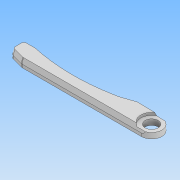
# Autodesk Inventor part: DoubleCrossBar
Saved by Autodesk Inventor 2021 (Build 250183000, 183)
## iProperties
Created: 2021-02-18
Part Number: DoubleCrossBar
Material: 一般
Document SubType Name: Modeling
Designer: kumagai
Density: 1 g/cm^3
Appearance: 既定
Author: kumagai
Autodesk Inventor part; units mm, degrees
ref_plane "YZ Plane" through (0, 0, 0) normal (1, 0, 0) x (0, 1, 0)
ref_plane "XZ Plane" through (0, 0, 0) normal (0, 1, 0) x (-1, 0, 0)
ref_plane "XY Plane" through (0, 0, 0) normal (0, 0, 1) x (1, 0, 0)
sketch "スケッチ1" plane through (0, 0, 0) normal (0, 1, 0) x (-1, 0, 0)
  line L0 (0, -94.2305) -> (0, 20.4332) projected
  line L1 (-15.3636, 0) -> (63.8106, 0) projected
  arc A0 (0, 4) -> (-0.1067, -3.9986) centre (0, 0) ccw
  line L2 (0, 4) -> (46.9019, 4)
  arc A1 (47.548, -2.5) -> (16.9578, -1.985) centre (30.98, -77.85) ccw
  line L3 (52.5, 2.5) -> (52.5, -2.5)
  line L4 (-0.1067, -3.9986) -> (9.3002, -4.2495)
  circle A2 centre (0, 0) radius 2.55
  line L5 (52.5, 2.5) -> (46.9019, 4)
  line L6 (52.5, -2.5) -> (47.548, -2.5)
  line L7 (9.3002, -4.2495) -> (14.9911, -2.3485)
  line L8 (14.9911, -2.3485) -> (16.9578, -1.985)
  dimension "d1" = 8
  dimension "d2" = 81.85
  dimension "d5" = 5.1
  dimension "d12" = 2.5
  dimension "d13" = 2.5
  dimension "d14" = 15
  dimension "d16" = 52.5
  dimension "d17" = 21.52
  dimension "d23" = 20
  dimension "d24" = 2
  dimension "d25" = 8
  dimension "d26" = 6
  dimension "d27" = 77.15
  constraints: 14 end point, 4 point on circle, 3 centre point, 3 tangent, 2 coincident, 2 horizontal, 1 point on line, 1 vertical
  measures "d1" diameter of A0
  measures "d2" distance from line of A1.centre L2
  measures "d5" diameter of A2
  measures "d12" distance between parallel lines of L6 L1
  measures "d13" distance from line of L1 L3.start
  measures "d14" angle of L2 L5
  measures "d16" distance between parallel lines of L3 L0
  measures "d17" distance from line of A1.centre L3
  measures "d23" angle of L4 L7
  measures "d24" distance of L7.end L8.end
  measures "d25" angle of L7 L8
  measures "d26" distance of L4.end L7.end
  measures "d27" radius of A1
extrude "押し出し1" add sketch "スケッチ1" along normal blind 3.2 contours L4 A0 L1 A2 L0 | L0 A2 L1 L3 L6 A1 L8 L7 L4 | L1 A0 L0 A2 | A2 L0 L2 L5 L3 L1
fillet "フィレット1" radius 1.5 6 edges at (-52.5, 1.6, 2.5) (-46.9019, 1.6, 4) (-52.5, 1.6, -2.5) (-47.548, 1.6, -2.5) (-9.3002, 1.6, -4.2495) (-14.9911, 1.6, -2.3485)
sketch "スケッチ2" plane through (0, 3.2, 0) normal (0, 1, 0) x (1, 0, 0)
  circle A0 centre (0, 0) radius 4.25
  dimension "d9" = 8.5
  constraints: 1 centre point, 1 coincident
  measures "d9" diameter of A0
extrude "押し出し2" cut sketch "スケッチ2" against normal blind 1
chamfer "面取り1" distance 0.5 distance2 2 10 edges at (-24.0703, 3.2, 4) (-46.9002, 3.2, 3.9872) (-49.2405, 3.2, 3.3734) (-52.19, 3.2, 2.2622) (-52.5, 3.2, 0.1745) (-52.0607, 3.2, -2.0607) (-49.3551, 3.2, -2.5) (-47.5498, 3.2, -2.4914) (-32.1984, 3.2, -0.7096) (-5.1824, 3.2, -4.1397) measured on face at (-49.3551, 3.2, -2) measured on face at (-51.7934, 3.2, 1.9578) measured on face at (-32.2063, 3.2, -0.2097) measured on face at (-52, 3.2, 0.1745) measured on face at (-5.1957, 3.2, -3.6399) measured on face at (-24.0703, 3.2, 3.5) measured on face at (-46.835, 3.2, 3.4914) measured on face at (-51.7071, 3.2, -1.7071) measured on face at (-49.111, 3.2, 2.8904) measured on face at (-47.6032, 3.2, -1.9943)
